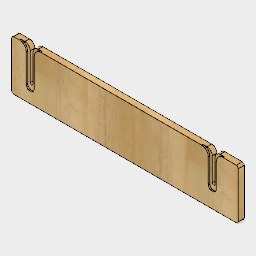
Parallel_Fraesanschlag_2_1_v7 (Autodesk Fusion 360 design; units mm, degrees)
Autodesk Fusion 360 part; units mm, degrees
sketch "Sketch1" plane through (0, 0, 0) normal (0, 0, 1) x (1, 0, 0)
  line L0 (6, 0) -> (674, 0)
  line L1 (680, 6) -> (680, 144)
  line L2 (0, 144) -> (0, 6)
  line L3 (52, 134) -> (52, 51)
  line L4 (60, 134) -> (60, 51)
  arc A0 (52, 51) -> (60, 51) centre (56, 51) ccw
  line L5 (598, 134) -> (598, 64)
  line L6 (606, 134) -> (606, 64)
  arc A1 (598, 64) -> (606, 64) centre (602, 64) ccw
  arc A2 (0, 6) -> (6, 0) centre (6, 6) ccw
  arc A3 (6, 150) -> (0, 144) centre (6, 144) ccw
  arc A4 (680, 144) -> (674, 150) centre (674, 144) ccw
  arc A5 (674, 0) -> (680, 6) centre (674, 6) ccw
  arc A6 (52, 134) -> (36, 150) centre (36, 134) ccw
  arc A7 (76, 150) -> (60, 134) centre (76, 134) ccw
  arc A8 (598, 134) -> (582, 150) centre (582, 134) ccw
  arc A9 (622, 150) -> (606, 134) centre (622, 134) ccw
  line L7 (622, 150) -> (674, 150)
  line L8 (76, 150) -> (582, 150)
  line L9 (36, 150) -> (6, 150)
  point P0 (680, 0)
  point P1 (0, 150)
  point P2 (52, 150)
  point P3 (60, 150)
  point P4 (598, 150)
  point P5 (606, 150)
  point P6 (44, 150)
  point P7 (68, 150)
  point P8 (590, 150)
  point P9 (614, 150)
  dimension "d1" = 680
  dimension "d2" = 150
  dimension "d3" = 99
  dimension "d4" = 52
  dimension "d5" = 99
  dimension "d6" = 60
  dimension "d7" = 86
  dimension "d8" = 598
  dimension "d9" = 86
  dimension "d10" = 606
  dimension "d11" = 6
  dimension "d12" = 16
  measures "d1" distance of origin P0
  measures "d2" distance of origin P1
  measures "d3" distance of P2 L3.end
  measures "d4" distance of L2 L3
  measures "d5" distance of P3 L4.end
  measures "d6" distance of L2 L4
  measures "d7" distance of P4 L5.end
  measures "d8" distance of L2 L5
  measures "d9" distance of P5 L6.end
  measures "d10" distance of L2 L6
  measures "d11" radius of A2
  measures "d12" radius of A6
extrude "Extrude1" add sketch "Sketch1" along normal blind 14
sketch "Sketch2" plane through (0, 0, 14) normal (0, 0, 1) x (1, 0, 0)
  arc A0 (52, 134) -> (36, 150) centre (36, 134) ccw
  line L0 (36, 150) -> (6, 150)
  arc A1 (6, 150) -> (0, 144) centre (6, 144) ccw
  line L1 (0, 144) -> (0, 6)
  arc A2 (0, 6) -> (6, 0) centre (6, 6) ccw
  line L2 (6, 0) -> (674, 0)
  arc A3 (674, 0) -> (680, 6) centre (674, 6) ccw
  line L3 (680, 6) -> (680, 144)
  arc A4 (680, 144) -> (674, 150) centre (674, 144) ccw
  line L4 (674, 150) -> (622, 150)
  arc A5 (622, 150) -> (606, 134) centre (622, 134) ccw
  line L5 (606, 134) -> (606, 64)
  arc A6 (598, 64) -> (606, 64) centre (602, 64) ccw
  line L6 (598, 64) -> (598, 134)
  arc A7 (598, 134) -> (582, 150) centre (582, 134) ccw
  line L7 (582, 150) -> (76, 150)
  arc A8 (76, 150) -> (60, 134) centre (76, 134) ccw
  line L8 (60, 134) -> (60, 51)
  arc A9 (52, 51) -> (60, 51) centre (56, 51) ccw
  line L9 (52, 51) -> (52, 134)
  line L10 (44, 130) -> (44, 45)
  line L11 (0, 144) -> (0, 6)
  line L12 (68, 130) -> (68, 45)
  arc A10 (44, 45) -> (68, 45) centre (56, 45) ccw
  line L13 (590, 130) -> (590, 58)
  line L14 (614, 130) -> (614, 58)
  arc A11 (590, 58) -> (614, 58) centre (602, 58) ccw
  line L15 (88, 150) -> (570, 150)
  line L16 (634, 150) -> (674, 150)
  arc A12 (88, 150) -> (68, 130) centre (88, 130) ccw
  line L17 (6, 150) -> (24, 150)
  arc A13 (44, 130) -> (24, 150) centre (24, 130) ccw
  arc A14 (590, 130) -> (570, 150) centre (570, 130) ccw
  arc A15 (634, 150) -> (614, 130) centre (634, 130) ccw
  point P0 (44, 150)
  point P1 (68, 150)
  point P2 (590, 150)
  point P3 (614, 150)
  dimension "d27" = 105
  dimension "d28" = 44
  dimension "d29" = 105
  dimension "d30" = 68
  dimension "d31" = 92
  dimension "d32" = 590
  dimension "d33" = 92
  dimension "d34" = 614
  dimension "d35" = 20
  dimension "d36" = 20
  dimension "d37" = 20
  dimension "d38" = 20
  measures "d27" distance of P0 L10.end
  measures "d28" distance of L10 L11
  measures "d29" distance of P1 L12.end
  measures "d30" distance of L11 L12
  measures "d31" distance of P2 L13.end
  measures "d32" distance of L11 L13
  measures "d33" distance of P3 L14.end
  measures "d34" distance of L11 L14
  measures "d35" radius of A12
  measures "d36" radius of A13
  measures "d37" radius of A14
  measures "d38" radius of A15
extrude "Extrude2" add sketch "Sketch2" along normal blind 4 contours L0 A1 L1 A2 L2 A3 L3 A4 L4 L7 L10 L11 L12 A10 L13 L14 A11 L15 L16 A12 L17 A13 A14 A15
